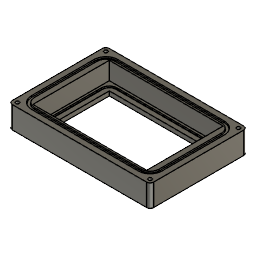
Base V2.1 (Autodesk Fusion 360 design; units mm, degrees)
part number: 2026-01-30-14-30-51-369
Autodesk Fusion 360 part; units mm, degrees
sketch "Sketch1" plane through (0, 0, 0) normal (0, 0, 1) x (1, 0, 0)
  line L0 (76, -55) -> (-76, -55)
  line L1 (-80, -51) -> (-80, 51)
  line L2 (-76, 55) -> (76, 55)
  line L3 (80, 51) -> (80, -51)
  line L4 (80, -55) -> (-80, 55) construction
  line L5 (-80, -55) -> (80, 55) construction
  arc A0 (-76, 55) -> (-80, 51) centre (-76, 51) ccw
  arc A1 (80, 51) -> (76, 55) centre (76, 51) ccw
  arc A2 (76, -55) -> (80, -51) centre (76, -51) ccw
  arc A3 (-80, -51) -> (-76, -55) centre (-76, -51) ccw
  circle A4 centre (-75, 50) radius 2
  line L6 (0, 55) -> (0, -55) construction
  line L7 (80, 0) -> (-80, 0) construction
  circle A5 centre (75, 50) radius 2
  circle A6 centre (75, -50) radius 2
  circle A7 centre (-75, -50) radius 2
  dimension "d1" = 160
  dimension "d2" = 110
  dimension "d26" = 4
  dimension "d27" = 4
  dimension "d28" = 4
  dimension "d29" = 4
  dimension "d30" = 4
  dimension "d31" = 5
  dimension "d32" = 5
  constraint horizontal L0
  constraint perpendicular L0 L1
  constraint parallel L0 L2
  constraint parallel L1 L3
  constraint coincident L4 origin
  constraint coincident L5 origin
  constraint coincident L4.end L2
  constraint coincident L4.end L1
  constraint tangent L2 A0
  constraint tangent L1 A0
  constraint coincident L5.end L3
  constraint coincident L5.end L2
  constraint tangent L3 A1
  constraint tangent L2 A1
  constraint coincident L4.start L3
  constraint coincident L4.start L0
  constraint tangent L3 A2
  constraint tangent L0 A2
  constraint coincident L5.start L1
  constraint coincident L5.start L0
  constraint tangent L1 A3
  constraint tangent L0 A3
  constraint midpoint L2 L6.start
  constraint midpoint L0 L6.end
  constraint midpoint L3 L7.start
  constraint midpoint L1 L7.end
  constraint symmetric A4 L6 A5
  constraint symmetric A4 L7 A7
  constraint symmetric L7 A5 A6
  measures "d1" distance of L4.end L5.end
  measures "d2" distance of L5.start L4.end
  measures "d26" radius of A0
  measures "d27" radius of A1
  measures "d28" radius of A2
  measures "d29" radius of A3
  measures "d30" diameter of A4
  measures "d31" distance of L2 A4.centre
  measures "d32" distance of L1 A4.centre
extrude "Extrude1" add sketch "Sketch1" along normal blind 25
sketch "Sketch2" plane through (0, 0, 25) normal (0, 0, 1) x (-1, 0, 0)
  line L0 (-76, -55) -> (76, -55)
  line L1 (80, -51) -> (80, 51)
  line L2 (76, 55) -> (-76, 55)
  line L3 (-80, 51) -> (-80, -51)
  line L4 (-64.4, 43.25) -> (64.4, 43.25)
  line L5 (64.4, 43.25) -> (64.4, -43.25)
  line L6 (64.4, -43.25) -> (-64.4, -43.25)
  line L7 (-64.4, -43.25) -> (-64.4, 43.25)
  line L8 (-64.4, 43.25) -> (64.4, -43.25) construction
  line L9 (64.4, 43.25) -> (-64.4, -43.25) construction
  arc A0 (76, -55) -> (80, -51) centre (76, -51) ccw
  arc A1 (80, 51) -> (76, 55) centre (76, 51) ccw
  arc A2 (-76, 55) -> (-80, 51) centre (-76, 51) ccw
  arc A3 (-80, -51) -> (-76, -55) centre (-76, -51) ccw
  circle A4 centre (75, 50) radius 2
  circle A5 centre (-75, 50) radius 2
  circle A6 centre (-75, -50) radius 2
  circle A7 centre (75, -50) radius 2
  dimension "d5" = 128.8
  dimension "d6" = 86.5
  constraint horizontal L4
  constraint perpendicular L4 L5
  constraint parallel L4 L6
  constraint parallel L5 L7
  constraint coincident L8 origin
  constraint coincident L9 origin
  measures "d5" distance of L5.end L6.end
  measures "d6" distance of L4.end L5.end
extrude "Extrude2" cut sketch "Sketch2" against normal blind 20 contours L4 L5 L6 L7
sketch "Sketch3" plane through (0, 0, 25) normal (0, 0, 1) x (-1, 0, 0)
  line L0 (64.4, 43.25) -> (64.4, -43.25)
  line L1 (64.4, -43.25) -> (-64.4, -43.25)
  line L2 (-64.4, -43.25) -> (-64.4, 43.25)
  line L3 (-64.4, 43.25) -> (64.4, 43.25)
  line L4 (-76, -55) -> (76, -55)
  line L5 (80, -51) -> (80, 51)
  line L6 (76, 55) -> (-76, 55)
  line L7 (-80, 51) -> (-80, -51)
  line L8 (-72.0964, 47.0964) -> (72.0964, 47.0964) construction
  line L9 (72.0964, 47.0964) -> (72.0964, -47.0964) construction
  line L10 (72.0964, -47.0964) -> (-72.0964, -47.0964) construction
  line L11 (-72.0964, -47.0964) -> (-72.0964, 47.0964) construction
  line L12 (-72.0964, 47.0964) -> (72.0964, -47.0964) construction
  line L13 (72.0964, 47.0964) -> (-72.0964, -47.0964) construction
  line L14 (70.6619, 35.3929) -> (70.6619, -35.3929)
  line L15 (60.3929, -45.6619) -> (-60.3929, -45.6619)
  line L16 (-70.6619, -35.3929) -> (-70.6619, 35.3929)
  line L17 (-70.6619, 45.6619) -> (70.6619, -45.6619) construction
  line L18 (70.6619, 45.6619) -> (-70.6619, -45.6619) construction
  line L19 (-60.3929, 48.5309) -> (60.3929, 48.5309)
  line L20 (73.5309, 35.3929) -> (73.5309, -35.3929)
  line L21 (60.3929, -48.5309) -> (-60.3929, -48.5309)
  line L22 (-73.5309, -35.3929) -> (-73.5309, 35.3929)
  line L23 (-73.5309, 48.5309) -> (73.5309, -48.5309) construction
  line L24 (73.5309, 48.5309) -> (-73.5309, -48.5309) construction
  arc A0 (60.3929, -45.6619) -> (70.6619, -35.3929) centre (60.3929, -35.3929) ccw
  arc A1 (60.3929, -48.5309) -> (73.5309, -35.3929) centre (60.3929, -35.3929) ccw
  line L25 (0, -55) -> (0, 55) construction
  line L26 (-80, 0) -> (80, 0) construction
  arc A2 (-70.6619, -35.3929) -> (-60.3929, -45.6619) centre (-60.3929, -35.3929) ccw
  arc A3 (-73.5309, -35.3929) -> (-60.3929, -48.5309) centre (-60.3929, -35.3929) ccw
  arc A4 (-60.3929, 45.6619) -> (-70.6619, 35.3929) centre (-60.3929, 35.3929) ccw
  arc A5 (-60.3929, 48.5309) -> (-73.5309, 35.3929) centre (-60.3929, 35.3929) ccw
  arc A6 (70.6619, 35.3929) -> (60.3929, 45.6619) centre (60.3929, 35.3929) ccw
  arc A7 (73.5309, 35.3929) -> (60.3929, 48.5309) centre (60.3929, 35.3929) ccw
  line L27 (-60.3929, 45.6619) -> (60.3929, 45.6619)
  arc A8 (76, -55) -> (80, -51) centre (76, -51) ccw
  arc A9 (80, 51) -> (76, 55) centre (76, 51) ccw
  arc A10 (-76, 55) -> (-80, 51) centre (-76, 51) ccw
  arc A11 (-80, -51) -> (-76, -55) centre (-76, -51) ccw
  circle A12 centre (75, 50) radius 2
  circle A13 centre (-75, 50) radius 2
  circle A14 centre (-75, -50) radius 2
  circle A15 centre (75, -50) radius 2
  dimension "d9" = 144.1928
  dimension "d15" = 94.1928
  dimension "d16" = 1.4345
  dimension "d17" = 1.4345
  dimension "d18" = 1.4345
  dimension "d19" = 1.4345
  dimension "d20" = 10.269
  dimension "d21" = 13.138
  constraint horizontal L8
  constraint perpendicular L8 L9
  constraint parallel L8 L10
  constraint parallel L9 L11
  constraint coincident L12 origin
  constraint coincident L13 origin
  constraint parallel L15 L27
  constraint parallel L14 L16
  constraint coincident L17 origin
  constraint coincident L18 origin
  constraint horizontal L19
  constraint perpendicular L19 L20
  constraint parallel L19 L21
  constraint parallel L20 L22
  constraint coincident L23 origin
  constraint coincident L24 origin
  constraint coincident L17.end L15
  constraint coincident L17.end L14
  constraint tangent L15 A0
  constraint tangent L14 A0
  constraint coincident L23.end L21
  constraint coincident L23.end L20
  constraint tangent L21 A1
  constraint tangent L20 A1
  constraint midpoint L4 L25.start
  constraint midpoint L6 L25.end
  constraint midpoint L7 L26.start
  constraint midpoint L5 L26.end
  constraint symmetric L15.start L25 L15.end
  constraint symmetric L14.end L25 L16.start
  constraint symmetric A0 L25 A2
  constraint symmetric L21.start L25 L21.end
  constraint symmetric L20.end L25 L22.start
  constraint symmetric A1 L25 A3
  constraint symmetric L15.start L26 A6.end
  constraint symmetric L14.end L26 L14.start
  constraint symmetric A0 L26 A6
  constraint symmetric L21.start L26 L19.end
  constraint symmetric L20.end L26 L20.start
  constraint symmetric A1 L26 A7
  constraint symmetric L26 L15.end A4.start
  constraint symmetric L26 L16.start L16.end
  constraint symmetric L26 A2 A4
  constraint symmetric L26 L21.end L19.start
  constraint symmetric L26 L22.start L22.end
  constraint symmetric L26 A3 A5
  measures "d9" distance of L8.start L8.end
  measures "d15" distance of L8 L10
  measures "d16" distance of L11 L16
  measures "d17" distance of L10 L15
  measures "d18" distance of L11 L22
  measures "d19" distance of L10 L21
  measures "d20" radius of A0
  measures "d21" radius of A1
extrude "Extrude3" cut sketch "Sketch3" against normal blind 1.424 contours L19 L20 L21 L22 A1 A3 A5 A7
draft "Draft1" angle 10 neutral plane through (0, 0, 23.576) pull (0, 0, 1) 16 faces at (-70.6619, -11.7976, 24.5253) (-67.8249, 42.4793, 24.0507) (-20.131, 45.6619, 24.5253) (67.4793, 42.8249, 24.0507) (70.6619, 11.7976, 24.5253) (67.8249, -42.4793, 24.0507) (20.131, -45.6619, 24.5253) (-64.2095, -44.9263, 24.5253) (-73.5309, -11.7976, 24.5253) (-70.7201, -43.5143, 24.0507) (20.131, -48.5309, 24.5253) (68.5143, -45.7201, 24.0507) (73.5309, 11.7976, 24.5253) (70.7201, 43.5143, 24.0507) (-20.131, 48.5309, 24.5253) (-71.0948, 43.0137, 24.0507)
sketch "Sketch4" plane through (0, 0, 5) normal (0, 0, 1) x (-1, 0, 0)
  line L0 (-64.4, -43.25) -> (64.4, -43.25)
  line L1 (64.4, -43.25) -> (64.4, 43.25)
  line L2 (64.4, 43.25) -> (-64.4, 43.25)
  line L3 (-64.4, 43.25) -> (-64.4, -43.25)
  line L4 (-54.4, 33.25) -> (54.4, 33.25)
  line L5 (54.4, 33.25) -> (54.4, -33.25)
  line L6 (54.4, -33.25) -> (-54.4, -33.25)
  line L7 (-54.4, -33.25) -> (-54.4, 33.25)
  line L8 (-54.4, 33.25) -> (54.4, -33.25) construction
  line L9 (54.4, 33.25) -> (-54.4, -33.25) construction
  dimension "d35" = 10
  dimension "d36" = 10
  constraint horizontal L4
  constraint perpendicular L4 L5
  constraint parallel L4 L6
  constraint parallel L5 L7
  constraint coincident L8 origin
  constraint coincident L9 origin
  measures "d35" distance of L3 L7
  measures "d36" distance of L0 L6
extrude "Extrude4" cut sketch "Sketch4" against normal blind 5 contours L4 L5 L6 L7
sketch "Sketch5" plane through (0, 0, 5) normal (0, 0, 1) x (-1, 0, 0)
  line L0 (54.4, 33.25) -> (54.4, -33.25)
  line L1 (54.4, -33.25) -> (-54.4, -33.25)
  line L2 (-54.4, -33.25) -> (-54.4, 33.25)
  line L3 (-54.4, 33.25) -> (54.4, 33.25)
  line L4 (-64.4, -43.25) -> (64.4, -43.25)
  line L5 (64.4, -43.25) -> (64.4, 43.25)
  line L6 (64.4, 43.25) -> (-64.4, 43.25)
  line L7 (-64.4, 43.25) -> (-64.4, -43.25)
  line L8 (-60.8342, 39.6842) -> (60.8342, 39.6842) construction
  line L9 (60.8342, 39.6842) -> (60.8342, -39.6842) construction
  line L10 (60.8342, -39.6842) -> (-60.8342, -39.6842) construction
  line L11 (-60.8342, -39.6842) -> (-60.8342, 39.6842) construction
  line L12 (-60.8342, 39.6842) -> (60.8342, -39.6842) construction
  line L13 (60.8342, 39.6842) -> (-60.8342, -39.6842) construction
  line L14 (59.7842, 31.4252) -> (59.7842, -31.4252)
  line L15 (52.5752, -38.6342) -> (-52.5752, -38.6342)
  line L16 (-59.7842, -31.4252) -> (-59.7842, 31.4252)
  line L17 (-57.1085, 36.9051) -> (59.7842, -38.6342) construction
  line L18 (57.4574, 36.3074) -> (-57.4574, -36.3074) construction
  line L19 (-52.8062, 40.6187) -> (52.8062, 40.6187)
  line L20 (61.8842, 31.5407) -> (61.8842, -31.5407)
  line L21 (52.8062, -40.6187) -> (-52.8062, -40.6187)
  line L22 (-61.8842, -31.5407) -> (-61.8842, 31.5407)
  line L23 (-58.9962, 38.7231) -> (61.8842, -40.6187) construction
  line L24 (59.3264, 38.1764) -> (-59.3264, -38.1764) construction
  arc A0 (52.5752, -38.6342) -> (59.7842, -31.4252) centre (52.5752, -31.4252) ccw
  arc A1 (52.8062, -40.6187) -> (61.8842, -31.5407) centre (52.8062, -31.5407) ccw
  line L25 (0, -43.25) -> (0, 43.25) construction
  line L26 (-64.4, 0) -> (64.4, 0) construction
  arc A2 (-59.7842, -31.4252) -> (-52.5752, -38.6342) centre (-52.5752, -31.4252) ccw
  arc A3 (-61.8842, -31.5407) -> (-52.8062, -40.6187) centre (-52.8062, -31.5407) ccw
  arc A4 (59.7842, 31.4252) -> (52.5752, 38.6342) centre (52.5752, 31.4252) ccw
  arc A5 (61.8842, 31.5407) -> (52.8062, 40.6187) centre (52.8062, 31.5407) ccw
  arc A6 (-52.5752, 38.6342) -> (-59.7842, 31.4252) centre (-52.5752, 31.4252) ccw
  arc A7 (-52.8062, 40.6187) -> (-61.8842, 31.5407) centre (-52.8062, 31.5407) ccw
  line L27 (-52.5752, 38.6342) -> (52.5752, 38.6342)
  dimension "d42" = 121.6684
  dimension "d43" = 79.3684
  dimension "d44" = 1.05
  dimension "d45" = 0.9345
  dimension "d46" = 1.05
  dimension "d47" = 1.05
  dimension "d48" = 7.209
  dimension "d49" = 9.078
  constraint horizontal L8
  constraint perpendicular L8 L9
  constraint parallel L8 L10
  constraint parallel L9 L11
  constraint coincident L12 origin
  constraint coincident L13 origin
  constraint parallel L15 L27
  constraint parallel L14 L16
  constraint coincident L17 origin
  constraint coincident L18 origin
  constraint horizontal L19
  constraint perpendicular L19 L20
  constraint parallel L19 L21
  constraint parallel L20 L22
  constraint coincident L23 origin
  constraint coincident L24 origin
  constraint coincident L17.end L15
  constraint coincident L17.end L14
  constraint tangent L15 A0
  constraint tangent L14 A0
  constraint coincident L23.end L21
  constraint coincident L23.end L20
  constraint tangent L21 A1
  constraint tangent L20 A1
  constraint midpoint L4 L25.start
  constraint midpoint L6 L25.end
  constraint midpoint L7 L26.start
  constraint midpoint L5 L26.end
  constraint symmetric L15.start L25 L15.end
  constraint symmetric L14.end L25 L16.start
  constraint symmetric A0 L25 A2
  constraint symmetric L21.start L25 L21.end
  constraint symmetric L20.end L25 L22.start
  constraint symmetric A1 L25 A3
  constraint symmetric L15.start L26 A4.end
  constraint symmetric L14.end L26 L14.start
  constraint symmetric A0 L26 A4
  constraint symmetric L21.start L26 L19.end
  constraint symmetric L20.end L26 L20.start
  constraint symmetric A1 L26 A5
  constraint symmetric L26 L15.end A6.start
  constraint symmetric L26 L16.start L16.end
  constraint symmetric L26 A2 A6
  constraint symmetric L26 L21.end L19.start
  constraint symmetric L26 L22.start L22.end
  constraint symmetric L26 A3 A7
  measures "d42" distance of L9 L11
  measures "d43" distance of L8 L10
  measures "d44" distance of L11 L22
  measures "d45" distance of L8 L19
  measures "d46" distance of L8 L27
  measures "d47" distance of L11 L16
  measures "d48" radius of A0
  measures "d49" radius of A1
extrude "Extrude5" cut sketch "Sketch5" against normal blind 1.6 contours L19 L20 L21 L22 A1 A3 A5 A7
equation "d9 = ( ORingPerimeter - 100 mm ) / 4 + 50 mm"
equation "ORingDiameter = 1.78 mm" comment "Diamter of the O ring"
equation "ORingInnerDiameter = 150 mm" comment "Inner diamter of the o ring bore"
equation "ORingPerimeter = 2 * 3.1412 * ( ( ORingInnerDiameter / 2 ) + ORingDiameter / 2 )"
equation "PanelWidth = 80 mm"
equation "PanelLength = 115 mm"
equation "d15 = ( ORingPerimeter - 100 mm ) / 4"
equation "d16 = ( ( ORingDiameter * 1.05 ) / 2 ) + 0.5 mm"
equation "d17 = ( ( ORingDiameter * 1.05 ) / 2 ) + 0.5 mm"
equation "d18 = ( ( ORingDiameter * 1.05 ) / 2 ) + 0.5 mm"
equation "d19 = ( ( ORingDiameter * 1.05 ) / 2 ) + 0.5 mm"
equation "d20 = ( ORingDiameter ) * 6 + ORingDiameter * 0.05 - 0.5 mm"
equation "d21 = ( ORingDiameter ) * 6 + ( ORingDiameter * 1.1 ) + 0.5 mm"
equation "d22 = -ORingDiameter * 0.8"
equation "ORing2Diameter = 2 mm" comment "Second O ring Diameter"
equation "ORing2InnerDiameter = 126 mm" comment "Inner diameter of the second O Ring"
equation "ORing2Perimeter = 2 * 3.1412 * ( ( ORing2InnerDiameter / 2 ) + ORing2Diameter / 2 )"
equation "d42 = ( ORing2Perimeter - 84.6 mm ) / 4 + 42.3 mm"
equation "d43 = ( ORing2Perimeter - 84.6 mm ) / 4"
equation "d44 = ( ORing2Diameter * 1.05 ) / 2"
equation "d45 = ( ORingDiameter * 1.05 ) / 2"
equation "d46 = ( ORing2Diameter * 1.05 ) / 2"
equation "d47 = ( ORing2Diameter * 1.05 ) / 2"
equation "d48 = ( ORingDiameter ) * 4 + ORingDiameter * 0.05 - 0.0 mm"
equation "d49 = ( ORingDiameter ) * 4 + ORingDiameter * 1.1 + 0 mm"
equation "d50 = -ORing2Diameter * 0.8"
